Autodesk Fusion 360 part; units mm, degrees
note: some values were not read from the file. Set by a fixed rule: which sketch regions a step uses.
(part 2 of 2)
sketch "Sketch28" plane through (0, 42.6, 0) normal (0, 1, 0) x (-1, 0, 0)
  line L0 (51.5, 0) -> (51.5, 10)
  line L1 (51.5, 10) -> (-67.5, 10)
  line L2 (-67.5, 10) -> (-67.5, 0)
  line L3 (-67.5, 0) -> (51.5, 0)
  line L4 (-57.4565, 8) -> (-24.05, 8)
  line L5 (-22.05, 6) -> (-22.05, 4)
  line L6 (-24.05, 2) -> (-57.4565, 2)
  line L7 (-59.4565, 4) -> (-59.4565, 6)
  line L8 (-3.575, 8) -> (3.575, 8)
  line L9 (5.575, 6) -> (5.575, 4)
  line L10 (3.575, 2) -> (-3.575, 2)
  line L11 (-5.575, 4) -> (-5.575, 6)
  line L12 (24.05, 8) -> (41.4565, 8)
  line L13 (43.4565, 6) -> (43.4565, 4)
  line L14 (41.4565, 2) -> (24.05, 2)
  line L15 (22.05, 4) -> (22.05, 6)
  arc A0 (-57.4565, 8) -> (-59.4565, 6) centre (-57.4565, 6) ccw
  arc A1 (-22.05, 6) -> (-24.05, 8) centre (-24.05, 6) ccw
  arc A2 (-24.05, 2) -> (-22.05, 4) centre (-24.05, 4) ccw
  arc A3 (-59.4565, 4) -> (-57.4565, 2) centre (-57.4565, 4) ccw
  arc A4 (-3.575, 8) -> (-5.575, 6) centre (-3.575, 6) ccw
  arc A5 (5.575, 6) -> (3.575, 8) centre (3.575, 6) ccw
  arc A6 (3.575, 2) -> (5.575, 4) centre (3.575, 4) ccw
  arc A7 (-5.575, 4) -> (-3.575, 2) centre (-3.575, 4) ccw
  arc A8 (24.05, 8) -> (22.05, 6) centre (24.05, 6) ccw
  arc A9 (43.4565, 6) -> (41.4565, 8) centre (41.4565, 6) ccw
  arc A10 (41.4565, 2) -> (43.4565, 4) centre (41.4565, 4) ccw
  arc A11 (22.05, 4) -> (24.05, 2) centre (24.05, 4) ccw
  point P0 (-20.05, 10)
  point P1 (20.05, 10)
  dimension "d256" = 2
  dimension "d257" = 2
  dimension "d258" = 2
  dimension "d259" = 37.4065
  dimension "d260" = 2
  dimension "d261" = 2
  dimension "d262" = 2
  dimension "d263" = 21.4065
  dimension "d264" = 2
  dimension "d265" = 11.15
  dimension "d266" = 5.575
  constraint horizontal L4
  constraint vertical L5
  constraint horizontal L6
  constraint vertical L7
  constraint horizontal L8
  constraint vertical L9
  constraint horizontal L10
  constraint vertical L11
  constraint horizontal L12
  constraint vertical L13
  constraint horizontal L14
  constraint vertical L15
  constraint tangent L7 A0
  constraint tangent L4 A0
  constraint tangent L4 A1
  constraint tangent L5 A1
  constraint equal A0 A1
  constraint tangent L5 A2
  constraint tangent L6 A2
  constraint equal A0 A2
  constraint tangent L6 A3
  constraint tangent L7 A3
  constraint equal A0 A3
  constraint tangent L11 A4
  constraint tangent L8 A4
  constraint tangent L8 A5
  constraint tangent L9 A5
  constraint equal A4 A5
  constraint tangent L9 A6
  constraint tangent L10 A6
  constraint equal A4 A6
  constraint tangent L10 A7
  constraint tangent L11 A7
  constraint equal A4 A7
  constraint tangent L15 A8
  constraint tangent L12 A8
  constraint tangent L12 A9
  constraint tangent L13 A9
  constraint equal A8 A9
  constraint tangent L13 A10
  constraint tangent L14 A10
  constraint equal A8 A10
  constraint tangent L14 A11
  constraint tangent L15 A11
  constraint equal A8 A11
  constraint horizontal A1.centre A4.centre
  constraint horizontal A2.centre A7.centre
  constraint horizontal A5.centre A8.centre
  constraint horizontal A6.centre A11.centre
  measures "d256" distance of L5 P0
  measures "d257" distance of L1 L4
  measures "d258" distance of L3 L6
  measures "d259" distance of L5 L7
  measures "d260" radius of A0
  measures "d261" radius of A4
  measures "d262" radius of A8
  measures "d263" distance of L13 L15
  measures "d264" distance of L15 P1
  measures "d265" distance of L9 L11
  measures "d266" distance of origin L9
extrude "Extrude32" cut sketch "Sketch28" against normal blind 7 contours L4 L5 L6 L7 A0 A1 A2 A3 | L8 L9 L10 L11 A4 A5 A6 A7 | L12 L13 L14 L15 A8 A9 A10 A11
sketch "Sketch29" plane through (0, -28.5, 0) normal (0, -1, 0) x (1, 0, 0)
  line L0 (-61.5, 0) -> (-61.5, 6.5)
  line L1 (-61.5, 6.5) -> (-72.5, 6.5)
  line L2 (-72.5, 6.5) -> (-72.5, 0)
  line L3 (-72.5, 0) -> (-61.5, 0)
  line L4 (-69.5, 4.5) -> (-62.5, 4.5)
  line L5 (-61.5, 3.5) -> (-61.5, 3)
  line L6 (-62.5, 2) -> (-69.5, 2)
  line L7 (-70.5, 3) -> (-70.5, 3.5)
  arc A0 (-69.5, 4.5) -> (-70.5, 3.5) centre (-69.5, 3.5) ccw
  arc A1 (-61.5, 3.5) -> (-62.5, 4.5) centre (-62.5, 3.5) ccw
  arc A2 (-62.5, 2) -> (-61.5, 3) centre (-62.5, 3) ccw
  arc A3 (-70.5, 3) -> (-69.5, 2) centre (-69.5, 3) ccw
  point P0 (-61.5, 6.5)
  point P1 (-59.5, 6.5)
  dimension "d270" = 2
  dimension "d271" = 2
  dimension "d272" = 2
  dimension "d273" = 1
  dimension "d274" = 2
  constraint horizontal L4
  constraint vertical L5
  constraint horizontal L6
  constraint vertical L7
  constraint tangent L7 A0
  constraint tangent L4 A0
  constraint tangent L4 A1
  constraint tangent L5 A1
  constraint equal A0 A1
  constraint tangent L5 A2
  constraint tangent L6 A2
  constraint equal A0 A2
  constraint tangent L6 A3
  constraint tangent L7 A3
  constraint equal A0 A3
  measures "d270" distance of L2 L7
  measures "d271" distance of L1 L4
  measures "d272" distance of L3 L6
  measures "d273" radius of A0
  measures "d274" distance of L5 P1
extrude "Extrude33" cut sketch "Sketch29" against normal blind 60 contours L0 L4 L5 L6 L7 A0 A1 A2 A3
equation "d2 = ( 145 / 2 ) * 1 mm"
equation "d4 = ( 57.1 / 2 ) * 1 mm"
equation "d82 = ( 57 / 2 ) * 1 mm"
equation "d153 = ( 3.5 / 2 ) * 1 mm"
equation "d161 = ( 4.85 / 2 ) * 1 mm + 2 mm"
equation "d162 = ( 4.85 / 2 ) * 1 mm + 2 mm"
equation "d178 = ( 7.087 / 2 ) * 1 mm + 2 mm"
equation "d179 = ( 7.087 / 2 ) * 1 mm + 2 mm"
equation "d208 = ( 36.1 / 2 ) * 1 mm"
equation "d215 = ( 4.85 / 2 ) * 1 mm + 2 mm"
equation "d216 = ( 4.85 / 2 ) * 1 mm + 2 mm"
equation "d221 = ( 4.85 / 2 ) * 1 mm + 2 mm"
equation "d222 = ( 4.85 / 2 ) * 1 mm + 2 mm"
equation "d230 = ( 36.1 / 2 ) * 1 mm"
equation "d251 = ( 11.15 / 2 ) * 1 mm"
equation "d266 = ( 11.15 / 2 ) * 1 mm"
